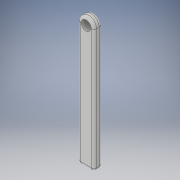
# Autodesk Inventor part: ручка
Saved by Autodesk Inventor 2019 (Build 230136000, 136)
## iProperties
Created: 2019-04-29
Part Number: ручка
Material: Типовые
Document SubType Name: Modeling
Designer: BarmanKaktus
Density: 1 g/cm^3
Appearance: По умолчанию
Author: BarmanKaktus
Autodesk Inventor part; units mm, degrees
ref_plane "YZ Plane" through (0, 0, 0) normal (1, 0, 0) x (0, 1, 0)
sketch "Эскиз1" plane through (0, 0, 0) normal (0, 0, 1) x (1, 0, 0)
  line L0 (0, 0) -> (-6, 0)
  line L1 (-6, 0) -> (-6, 47)
  line L2 (-6, 47) -> (0, 47)
  line L3 (0, 47) -> (0, 0)
  dimension "d0" = 6
  dimension "d1" = 47
  constraints: 8 end point, 2 parallel, 1 horizontal, 1 perpendicular
  measures "d0" distance of L1.end L2.end
  measures "d1" distance of L0.end L1.end
extrude "Выдавливание1" add sketch "Эскиз1" along normal blind 3
fillet "Сопряжение1" radius 1 2 edges at (0, 0, 1.5) (-6, 0, 1.5)
ref_plane "РабПлоскость1" through (0, 0, 3) normal (0, 0, 1) x (1, 0, 0)
sketch "Эскиз3" plane through (0, 0, 3) normal (0, 0, 1) x (1, 0, 0)
  line L0 (0, 47) -> (-6, 47) projected
  circle A0 centre (-3, 47) radius 3
  point P0 (0, 0)
  dimension "d6" = 6
  constraints: 1 centre point, 1 midpoint
  measures "d6" diameter of A0
extrude "Выдавливание2" add sketch "Эскиз3" against normal blind 3
ref_plane "РабПлоскость2" through (0, 0, 3) normal (0, 0, 1) x (1, 0, 0)
sketch "Эскиз4" plane through (0, 0, 3) normal (0, 0, 1) x (1, 0, 0)
  circle A0 centre (-3, 47) radius 1.75
  point P0 (0, 0)
  dimension "d10" = 3.5
  constraints: 1 centre point
  measures "d10" diameter of A0
extrude "Выдавливание3" cut sketch "Эскиз4" against normal through all
fillet "Сопряжение2" radius 1 12 edges at (-0.2929, 0.2929, 3) (0, 24, 3) (-3, 50, 3) (-6, 24, 3) (-5.7071, 0.2929, 3) (-3, 0, 3) (-5.7071, 0.2929, 0) (-6, 24, 0) (-3, 50, 0) (0, 24, 0) (-0.2929, 0.2929, 0) (-3, 0, 0)
